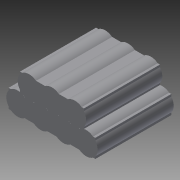
# Autodesk Inventor part: pololu_batterie_8p4v
Saved by Autodesk Inventor 2014 SP1 (Build 180222100, 222)
## iProperties
Created: 2015-08-03
Part Number: pololu_batterie_8p4v
Material: Générique
Document SubType Name: Modeling
Designer: astralien3000
Density: 1 g/cm^3
Appearance: Par défaut
Author: astralien3000
Autodesk Inventor part; units mm, degrees
ref_plane "YZ Plane" through (0, 0, 0) normal (1, 0, 0) x (0, 1, 0)
ref_plane "XZ Plane" through (0, 0, 0) normal (0, 1, 0) x (-1, 0, 0)
ref_plane "XY Plane" through (0, 0, 0) normal (0, 0, 1) x (1, 0, 0)
sketch "Esquisse1" plane through (0, 0, 0) normal (0, 1, 0) x (-1, 0, 0)
  line L0 (-22.5, 0) -> (22.5, 0)
  circle A0 centre (-22.5, 0) radius 7.5
  circle A1 centre (-7.5, 0) radius 7.5
  circle A2 centre (22.5, 0) radius 7.5
  circle A3 centre (7.5, 0) radius 7.5
  line L1 (-15, 12.9904) -> (15, 12.9904)
  circle A4 centre (-15, 12.9904) radius 7.5
  circle A5 centre (0, 12.9904) radius 7.5
  circle A6 centre (15, 12.9904) radius 7.5
  line L2 (-28.5, 6) -> (28.5, 6)
  line L3 (28.5, 6) -> (28.5, -6)
  line L4 (28.5, -6) -> (-28.5, -6)
  line L5 (-28.5, -6) -> (-28.5, 6)
  line L6 (21, 6.9904) -> (-21, 6.9904)
  line L7 (-21, 6.9904) -> (-21, 18.9904)
  line L8 (-21, 18.9904) -> (21, 18.9904)
  line L9 (21, 18.9904) -> (21, 6.9904)
  point P0 (0, 0)
  point P1 (0, 0)
  dimension "d0" = 15
  dimension "d1" = 15
  dimension "d2" = 15
  dimension "d3" = 15
  dimension "d4" = 15
  dimension "d5" = 15
  dimension "d6" = 15
  dimension "d7" = 12
  dimension "d8" = 6
  dimension "d9" = 12
  dimension "d10" = 6
  dimension "d11" = 6
  dimension "d12" = 6
  dimension "d13" = 6
  dimension "d14" = 6
  constraints: 20 end point, 7 centre point, 7 equal radius, 5 coincident, 5 parallel, 3 horizontal, 2 midpoint, 2 perpendicular, 2 point on line
  measures "d0" diameter of A4
  measures "d1" diameter of A5
  measures "d2" diameter of A6
  measures "d3" diameter of A0
  measures "d4" diameter of A1
  measures "d5" diameter of A3
  measures "d6" diameter of A2
  measures "d7" distance between parallel lines of L6 L8
  measures "d8" distance between parallel lines of L6 L1
  measures "d9" distance between parallel lines of L2 L4
  measures "d10" distance between parallel lines of L0 L4
  measures "d11" distance from line of L0.start L5
  measures "d12" distance from line of L0.end L3
  measures "d13" distance from line of L1.end L9
  measures "d14" distance from line of L1.start L7
extrude "Extrusion1" add sketch "Esquisse1" along normal blind 50 contours A1 L2 L0 | A0 L4 L5 L2 | A1 L4 A0 | A0 L2 A4 A1 | L0 A1 L4 | A3 L2 L0 | A3 L4 A1 | A1 L2 A5 A3 | L0 A3 L4 | L2 A0 L7 L6 | A0 L4 | A1 L6 L2 | L4 A1 | A3 L2 A6 A2 | A2 L2 L3 L4 | A2 L4 A3 | A3 L6 L2 | L4 A3 | A4 L6 L2 | A0 L5 L2 | L2 A4 | L4 L5 A0 | A2 L6 L9 L2 | L4 A2 | A5 L6 L2 | L2 A5 | L6 L7 A0 | A0 L7 A4 L6 | A4 L7 L8 L6 | L5 A0 | L6 A4 A5 A1 | A1 L6 | A6 L2 L6 | A6 L2 | L2 L3 A2 | A2 L3 L4 | A5 L1 L6 | L6 A5 A6 A3 | A3 L6 | A4 L7 | A5 L8 L1 | A4 L8 A5 | L6 A6 L9 A2 | A2 L9 L6 | L6 A6 L8 L9 | A2 L3 | A5 L8 A6 | L7 L8 A4 | L8 A4 | A5 L8 | L9 A6 | A6 L8 | A6 L8 L9
equation "\"d1\" = d0"
equation "\"d3\" = d0"
equation "\"d4\" = d3"
equation "\"d5\" = d3"
equation "\"d6\" = d3"
equation "\"d8\" = 0.5 * d7"
equation "\"d10\" = 0.5 * d9"
equation "\"d11\" = d10"
equation "\"d12\" = d10"
equation "\"d13\" = d8"
equation "\"d14\" = d8"
